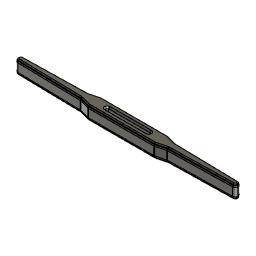
NG_1_CAD (Autodesk Fusion 360 design; units mm, degrees)
Autodesk Fusion 360 part; units mm, degrees
sketch "Sketch1" plane through (0, 0, 0) normal (0, 0, 1) x (1, 0, 0)
  line L0 (0, 1.9996) -> (0, 11.9996) construction
  line L1 (-80, 5) -> (80, 5) construction
  line L2 (-31.4641, 8) -> (-24, 10)
  line L3 (-24, 10) -> (0, 10)
  line L4 (-80, 5) -> (-80, 7)
  line L5 (-80, 7) -> (-31.4641, 8)
  line L6 (24, 10) -> (0, 10)
  line L7 (31.4641, 8) -> (24, 10)
  line L8 (80, 7) -> (31.4641, 8)
  line L9 (80, 5) -> (80, 7)
  line L10 (-80, 5) -> (-80, 3)
  line L11 (-80, 3) -> (-31.4641, 2)
  line L12 (-31.4641, 2) -> (-24, 0)
  line L13 (-24, 0) -> (0, 0)
  line L14 (24, 0) -> (0, 0)
  line L15 (31.4641, 2) -> (24, 0)
  line L16 (80, 3) -> (31.4641, 2)
  line L17 (80, 5) -> (80, 3)
  arc A0 (-15, 6) -> (-15, 4) centre (-15, 5) ccw
  arc A1 (15, 4) -> (15, 6) centre (15, 5) ccw
  line L18 (15, 6) -> (-15, 6)
  line L19 (-15, 4) -> (15, 4)
  line L20 (-15, 6) -> (15, 4) construction
  line L21 (15, 6) -> (-15, 4) construction
  point P0 (0, 5)
  point P1 (-80, 5)
  point P2 (0, 5)
  dimension "d4" = 2
  dimension "d9" = 160
  dimension "d10" = 10
  dimension "d11" = 4
  dimension "d12" = 48
  dimension "d13" = 6
  dimension "d14" = 165
  dimension "d25" = 30
  constraint midpoint L1 P2
  constraint coincident P1 L1.start
  constraint perpendicular L1 L4
  constraint symmetric L0 L2.start L7.start
  constraint symmetric L0 L2.end L6.start
  constraint symmetric L0 L3.end L6.end
  constraint symmetric L0 P1 L1.end
  constraint symmetric L0 L4.end L8.start
  constraint symmetric L1 L2.start L11.end
  constraint symmetric L1 L2.end L12.end
  constraint symmetric L1 L3.end L13.end
  constraint symmetric L1 P1 L4.start
  constraint symmetric L1 L4.end L10.end
  constraint symmetric L1 L6.start L14.start
  constraint symmetric L1 L7.start L15.start
  constraint symmetric L1 L8.start L16.start
  constraint symmetric L1 L9.start L17.start
  constraint coincident L3 L6.end
  constraint coincident L3.end L6.end
  constraint coincident L13.end L14.end
  constraint horizontal L3
  constraint symmetric L0 A0.start A1.end
  constraint symmetric L0 A0.end A1.start
  constraint symmetric L0 A0 A1
  constraint tangent A0 L18
  constraint tangent A1 L19
  constraint midpoint L21 P2
  constraint coincident P2 P0
  measures "d4" distance of A0.start A0.end
  measures "d9" distance of L4 L9
  measures "d10" distance of L3 L13
  measures "d11" distance of L4.end L10.end
  measures "d12" distance of L12.end L14.start
  measures "d13" distance of L7.start L15.start
  measures "d14" angle of L6 L7
  measures "d25" distance of A0.end A1.start
extrude "Extrude1" add sketch "Sketch1" along normal blind 10
fillet "Fillet2" radius 2 12 edges at (-31.4641, 2, 5) (-24, 0, 5) (24, 0, 5) (31.4641, 2, 5) (31.4641, 8, 5) (24, 10, 5) (80, 7, 5) (80, 3, 5) (-24, 10, 5) (-31.4641, 8, 5) (-80, 7, 5) (-80, 3, 5)
chamfer "Chamfer1" distance 1 angle 45 1 faces at (47.1513, 4.3199, 10)
chamfer "Chamfer2" distance 1 angle 45 1 faces at (47.1513, 4.3199, 0)
chamfer "Chamfer3" distance 0.5 angle 45 1 faces at (-80, 4.9864, 3.6667)
chamfer "Chamfer4" distance 0.5 angle 45 1 faces at (80, 4.9864, 3.8333)
